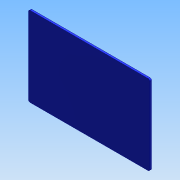
# Autodesk Inventor part: Paper-holder
Saved by Autodesk Inventor 2016 (Build 200138000, 138)
## iProperties
Created: 2015-10-22
Part Number: Paper-holder
Material: Generic
Document SubType Name: Modeling
Designer: Openlab
Density: 1 g/cm^3
Appearance: Blue - Wall Paint - Glossy
Author: Openlab
Autodesk Inventor part; units mm, degrees
ref_plane "YZ Plane" through (0, 0, 0) normal (1, 0, 0) x (0, 1, 0)
ref_plane "XZ Plane" through (0, 0, 0) normal (0, 1, 0) x (-1, 0, 0)
ref_plane "XY Plane" through (0, 0, 0) normal (0, 0, 1) x (1, 0, 0)
sketch "Sketch1" plane through (0, 0, 0) normal (0, 1, 0) x (-1, 0, 0)
  line L0 (145.7328, 113.0172) -> (-204.2672, 113.0172)
  line L1 (-204.2672, 113.0172) -> (-204.2672, -116.9828)
  line L2 (-204.2672, -116.9828) -> (145.7328, -116.9828)
  line L3 (145.7328, -116.9828) -> (145.7328, 113.0172)
  point P0 (0, 0)
  dimension "d0" = 230
  dimension "d1" = 350
  constraints: 8 end point, 2 parallel, 1 horizontal, 1 perpendicular
  measures "d0" distance of L2.end L0.start
  measures "d1" distance of L0.start L0.end
extrude "Extrusion1" add sketch "Sketch1" along normal blind 5
fillet "Fillet1" radius 5 4 edges at (204.2672, 2.5, 113.0172) (-145.7328, 2.5, 113.0172) (204.2672, 2.5, -116.9828) (-145.7328, 2.5, -116.9828)
body "Solid1"
